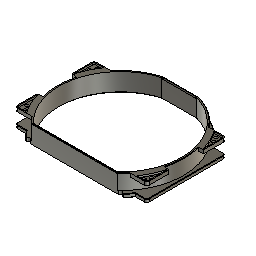
NH-D15 Spacer v9 (Autodesk Fusion 360 design; units mm, degrees)
Autodesk Fusion 360 part; units mm, degrees
sketch "Core" plane through (0, 0, 0) normal (0, 0, 1) x (1, 0, 0)
  line L0 (-49.3785, -52.4) -> (0, -52.4)
  line L1 (0, 69) -> (-20.567, 69)
  line L2 (0, 67) -> (-20.2731, 67)
  line L3 (0, -50) -> (-48.9898, -50)
  arc A0 (-20.2731, 67) -> (-48.9898, -50) centre (0, 0) ccw
  arc A1 (-20.567, 69) -> (-49.3785, -52.4) centre (0, 0) ccw
  line L4 (0, -50) -> (0, 0)
  line L5 (0, 0) -> (0, 67)
  line L6 (0, 67) -> (0, 69)
  line L7 (0, -50) -> (0, -52.4)
  line L8 (0, 69) -> (20.567, 69)
  arc A2 (49.3785, -52.4) -> (20.567, 69) centre (0, 0) ccw
  line L9 (49.3785, -52.4) -> (0, -52.4)
  line L10 (0, 67) -> (20.2731, 67)
  arc A3 (48.9898, -50) -> (20.2731, 67) centre (0, 0) ccw
  line L11 (0, -50) -> (48.9898, -50)
  dimension "d8" = 70
  dimension "d9" = 72
  dimension "d27" = 2
  dimension "d28" = 2.4
  dimension "d29" = 67
  dimension "d30" = 50
  constraint coincident A0.centre A1.centre
  constraint horizontal L3
  constraint horizontal L1
  constraint horizontal L2
  constraint horizontal L0
  constraint vertical L5
  constraint vertical L4
  constraint perpendicular L2 L6
  constraint perpendicular L0 L7
  constraint symmetric L3.start L5 L4.start
  constraint symmetric L0.start L5 A2.start
  constraint symmetric L3.end L5 A3.start
  constraint symmetric L1.end L5 L8.end
  constraint symmetric L2.start L5 L6.start
  constraint symmetric L2.end L5 L10.end
  constraint symmetric L0.end L5 L7.end
  constraint symmetric L1.start L5 L6.end
  constraint symmetric A0 L5 A3
  constraint symmetric A1 L5 A2
  measures "d8" radius of A0
  measures "d9" radius of A1
  measures "d27" distance of L1 L2
  measures "d28" distance of L0 L3
  measures "d29" vertical distance of L2.start A0.centre
  measures "d30" vertical distance of L3.start A0.centre
extrude "Extrude1" add sketch "Core" along normal blind 21 contours L0 L1 L2 L3 A0 A1 L6 L7 | L6 L7 L8 A2 L9 L10 A3 L11
sketch "Base" plane through (0, 0, 0) normal (0, 0, 1) x (1, 0, 0)
  line L0 (-31.3986, 69.7594) -> (0, 69.7594)
  line L1 (-72, 45) -> (-61.8648, 45)
  line L2 (-50.5025, -52.4) -> (-49.3785, -52.4)
  line L3 (-54.4975, -52.4) -> (-55.7359, -52.4)
  line L4 (-75, 42) -> (-75, -42)
  line L5 (-72, -45) -> (-61.8648, -45)
  line L6 (0, 0) -> (0, 67)
  line L7 (0, 69) -> (-20.567, 69)
  arc A0 (-20.567, 69) -> (-49.3785, -52.4) centre (0, 0) ccw
  line L8 (0, 69) -> (0, 69.7594)
  circle A1 centre (-52.5, 52.5) radius 2
  arc A2 (-21.8524, 73.3125) -> (-52.4647, -55.675) centre (0, 0) ccw
  circle A3 centre (-52.5, 52.5) radius 4.5
  circle A4 centre (-52.5, -52.5) radius 2
  arc A5 (-72, 45) -> (-75, 42) centre (-72, 42) ccw
  arc A6 (-75, -42) -> (-72, -45) centre (-72, -42) ccw
  arc A7 (49.3785, -52.4) -> (20.567, 69) centre (0, 0) ccw
  arc A8 (52.4647, -55.675) -> (21.8524, 73.3125) centre (0, 0) ccw
  line L9 (54.4975, -52.4) -> (55.7359, -52.4)
  line L10 (75, 42) -> (75, -42)
  line L11 (72, -45) -> (61.8648, -45)
  circle A9 centre (52.5, 52.5) radius 4.5
  arc A10 (75, 42) -> (72, 45) centre (72, 42) ccw
  line L12 (50.5025, -52.4) -> (49.3785, -52.4)
  circle A11 centre (52.5, 52.5) radius 2
  line L13 (72, 45) -> (61.8648, 45)
  circle A12 centre (52.5, -52.5) radius 2
  arc A13 (72, -45) -> (75, -42) centre (72, -42) ccw
  line L14 (0, 69) -> (20.567, 69)
  line L15 (31.3986, 69.7594) -> (0, 69.7594)
  point P0 (0, 67)
  dimension "d31" = 0.7594
  dimension "d40" = 75
  dimension "d43" = 4
  dimension "d44" = 52.5
  dimension "d45" = 52.5
  dimension "d46" = 4.5
  dimension "d47" = 9
  dimension "d64" = 4
  dimension "d65" = 52.5
  dimension "d66" = 52.5
  dimension "d67" = 90
  dimension "d69" = 45
  dimension "d71" = 84
  dimension "d72" = 42
  constraint coincident L7.start L8.start
  constraint perpendicular L0 L8
  constraint parallel L0 L7
  constraint horizontal L1
  constraint vertical L4
  constraint horizontal L2
  constraint horizontal L3
  constraint collinear L2 L3
  constraint parallel L1 L5
  constraint coincident A2 L0.start
  constraint concentric A1 A3
  constraint coincident A2 L1.end
  constraint coincident A2 L5.end
  constraint coincident L3.end A2
  constraint tangent L4 A5
  constraint tangent L5 A6
  constraint tangent L4 A6
  constraint tangent L1 A5
  constraint symmetric L4.start L6 L10.start
  constraint symmetric L4.end L6 L10.end
  constraint symmetric L1.start L6 A10.end
  constraint symmetric L2.start L6 L12.start
  constraint symmetric L5.start L6 L11.start
  constraint symmetric L3.start L6 L9.start
  constraint symmetric L0.end L6 L8.end
  constraint symmetric L3.end L6 L9.end
  constraint symmetric L6 L7.start L8.start
  constraint symmetric L6 L7.end A7.end
  constraint symmetric L6 L2.end A7.start
  constraint symmetric L6 A0 A7
  constraint symmetric L6 A1 A11
  constraint symmetric L6 A2.end A8.start
  constraint symmetric L6 A2.start A8.end
  constraint symmetric L6 A2 A8
  constraint symmetric L6 L0.start L15.start
  constraint symmetric L6 A3 A9
  constraint symmetric L6 L1.end L13.end
  constraint symmetric L6 L5.end L11.end
  constraint symmetric L6 A4 A12
  constraint symmetric L6 A5 A10
  constraint symmetric L6 A6 A13
  measures "d31" distance of L0 L7
  measures "d40" distance of L4 L6
  measures "d43" diameter of A1
  measures "d44" distance of L6 A1.centre
  measures "d45" vertical distance of L6.start A1.centre
  measures "d47" diameter of A3
  measures "d64" diameter of A4
  measures "d65" horizontal distance of L6.start A4.centre
  measures "d66" vertical distance of L6.start A4.centre
  measures "d67" distance of L1 L5
  measures "d69" distance of L6.start L1
  measures "d71" distance of L4.start L4.end
  measures "d72" vertical distance of L4.start L6.start
extrude "Extrude2" add sketch "Base" along normal blind 4 contours L0 L7 A0 L8 A2 A3 | L8 A7 A8 A9 L14 L15 | A0 A2 A3 | A2 A3 | L2 L3 L4 A0 A2 A3 A4 | A8 A9 | A7 A8 A9 | L1 L4 A2 A5 | A7 A8 L9 L10 A9 L12 A12 | A8 L10 A10 L13 | L4 L5 A2 A6 | A8 L10 L11 A13
ref_plane "WorkPlane3" through (0, 0, 21) normal (0, 0, 1) x (1, 0, 0)
sketch "Top" plane through (0, 0, 21) normal (0, 0, 1) x (1, 0, 0)
  line L0 (-73.9, 42) -> (-73.9, 20.9955)
  circle A0 centre (-70.9, 35.5) radius 1.8
  circle A1 centre (-67.9, 41) radius 1.8
  line L1 (-75, 20) -> (-69.4423, 19.02)
  line L2 (-73.9, 20.9955) -> (-73.5786, 20.9388)
  line L3 (-72, 43.9) -> (-62.8, 43.9)
  line L4 (-62.8, 43.9) -> (-62.8, 43.6854)
  line L5 (0, 0) -> (-10, 0)
  line L6 (-72, 45) -> (-61.8648, 45)
  arc A2 (-72, 45) -> (-75, 42) centre (-72, 42) ccw
  line L7 (-75, 42) -> (-75, -42)
  line L8 (-75, 20) -> (-75, 42)
  line L9 (-72, 45) -> (-56.205, 45)
  arc A3 (-21.8524, 73.3125) -> (-52.4647, -55.675) centre (0, 0) ccw
  arc A4 (-20.567, 69) -> (-49.3785, -52.4) centre (0, 0) ccw
  arc A5 (-72, 43.9) -> (-73.9, 42) centre (-72, 42) ccw
  arc A6 (-62.8, 43.6853) -> (-73.5786, 20.9388) centre (0, 0) ccw
  arc A7 (-56.205, 45) -> (-69.4423, 19.02) centre (0, 0) ccw
  line L10 (0, 0) -> (0, 67)
  line L11 (-75, -20) -> (-75, -42)
  line L12 (-73.9, -20.9955) -> (-73.5786, -20.9388)
  line L13 (-72, -43.9) -> (-62.8, -43.9)
  line L14 (-62.8, -43.9) -> (-62.8, -43.6853)
  arc A8 (-73.9, -42) -> (-72, -43.9) centre (-72, -42) ccw
  circle A9 centre (-67.9, -41) radius 1.8
  line L15 (-72, -45) -> (-61.8648, -45)
  circle A10 centre (-70.9, -35.5) radius 1.8
  line L16 (-75, -20) -> (-69.4423, -19.02)
  arc A11 (-73.5786, -20.9388) -> (-62.8, -43.6853) centre (0, 0) ccw
  line L17 (-72, -45) -> (-56.205, -45)
  arc A12 (-69.4423, -19.02) -> (-56.205, -45) centre (0, 0) ccw
  arc A13 (-75, -42) -> (-72, -45) centre (-72, -42) ccw
  line L18 (-73.9, -42) -> (-73.9, -20.9955)
  line L19 (62.8, -43.9) -> (62.8, -43.6853)
  circle A14 centre (67.9, 41) radius 1.8
  line L20 (73.9, -20.9955) -> (73.5786, -20.9388)
  line L21 (75, -20) -> (69.4423, -19.02)
  arc A15 (62.8, -43.6853) -> (73.5786, -20.9388) centre (0, 0) ccw
  line L22 (73.9, -42) -> (73.9, -20.9955)
  line L23 (72, -45) -> (56.205, -45)
  line L24 (73.9, 20.9955) -> (73.5786, 20.9388)
  arc A16 (73.5786, 20.9388) -> (62.8, 43.6853) centre (0, 0) ccw
  line L25 (72, -43.9) -> (62.8, -43.9)
  circle A17 centre (67.9, -41) radius 1.8
  line L26 (72, 43.9) -> (62.8, 43.9)
  arc A18 (75, 42) -> (72, 45) centre (72, 42) ccw
  line L27 (72, 45) -> (56.205, 45)
  arc A19 (73.9, 42) -> (72, 43.9) centre (72, 42) ccw
  arc A20 (72, -45) -> (75, -42) centre (72, -42) ccw
  line L28 (75, -20) -> (75, -42)
  arc A21 (56.205, -45) -> (69.4423, -19.02) centre (0, 0) ccw
  arc A22 (72, -43.9) -> (73.9, -42) centre (72, -42) ccw
  arc A23 (69.4423, 19.02) -> (56.205, 45) centre (0, 0) ccw
  line L29 (72, 45) -> (61.8648, 45)
  line L30 (62.8, 43.9) -> (62.8, 43.6853)
  line L31 (73.9, 42) -> (73.9, 20.9955)
  circle A24 centre (70.9, -35.5) radius 1.8
  line L32 (75, 20) -> (69.4423, 19.02)
  circle A25 centre (70.9, 35.5) radius 1.8
  line L33 (72, -45) -> (61.8648, -45)
  line L34 (75, 20) -> (75, 42)
  point P0 (-72, 41.9955)
  point P1 (-75, -42)
  point P2 (-72, -41.9955)
  point P3 (75, -42)
  point P4 (75, -42)
  point P5 (75, 42)
  point P6 (72, -41.9955)
  point P7 (72, 41.9955)
  dimension "d76" = 22
  dimension "d77" = 100
  dimension "d78" = -1.1
  dimension "d79" = 2.9
  dimension "d80" = 3
  dimension "d81" = 8.4
  dimension "d82" = 6
  dimension "d84" = 0.3263
  dimension "d85" = 3.6
  dimension "d86" = 3.6
  dimension "d89" = 9.2
  constraint coincident A2.end L7.start
  constraint tangent A2 L8
  constraint coincident L6.start A2.start
  constraint tangent A2 L9
  constraint perpendicular L8 L9
  constraint coincident A4 L9.end
  constraint coincident A4 L1.end
  constraint parallel L1 L2
  constraint parallel L0 L8
  constraint parallel L3 L9
  constraint tangent L3 A5
  constraint tangent L0 A5
  constraint perpendicular L3 L4
  constraint coincident A3 A6.start
  constraint coincident A3 L2.end
  constraint symmetric P0 L5 P2
  constraint symmetric L5 L3.start L13.start
  constraint symmetric L3.end L5 L13.end
  constraint symmetric L0.end L5 L12.start
  constraint symmetric L1.start L5 L11.start
  constraint symmetric L5 L0.start A8.start
  constraint symmetric A0 L5 A10
  constraint symmetric A1 L5 A9
  constraint symmetric L5 L6.start L15.start
  constraint symmetric L5 L6.end L15.end
  constraint symmetric L5 A2.end P1
  constraint symmetric L5 A2 A13
  constraint symmetric L5 L9.end L17.end
  constraint symmetric L5 L1.end L16.end
  constraint symmetric L5 A5 A8
  constraint symmetric L5 A6.start L14.end
  constraint symmetric L5 L2.end L12.end
  constraint symmetric L5 A6 A11
  constraint symmetric L5 A7 A12
  constraint symmetric P0 L10 P7
  constraint symmetric L3.start L10 L26.start
  constraint symmetric L3.end L10 L26.end
  constraint symmetric L0.end L10 L24.start
  constraint symmetric L1.start L10 L32.start
  constraint symmetric L0.start L10 A19.start
  constraint symmetric A0 L10 A25
  constraint symmetric A1 L10 A14
  constraint symmetric L6.start L10 A18.end
  constraint symmetric L6.end L10 L29.end
  constraint symmetric A2.end L10 P5
  constraint symmetric A2 L10 A18
  constraint symmetric P1 L10 P4
  constraint symmetric L9.end L10 L27.end
  constraint symmetric L1.end L10 A23.start
  constraint symmetric A5 L10 A19
  constraint symmetric A6.start L10 A16.end
  constraint symmetric L2.end L10 L24.end
  constraint symmetric A6 L10 A16
  constraint symmetric A7 L10 A23
  constraint symmetric L10 P1 P4
  constraint symmetric L10 L15.start L23.start
  constraint symmetric L10 L13.end L19.start
  constraint symmetric L10 L13.start L25.start
  constraint symmetric L10 L12.start L20.start
  constraint symmetric L10 L11.start L21.start
  constraint symmetric L10 A8.start L22.start
  constraint symmetric L10 L15.end L33.end
  constraint symmetric L10 L14.end L19.end
  constraint symmetric L10 L17.end L23.end
  constraint symmetric L10 P2 P6
  constraint symmetric L10 L12.end L20.end
  constraint symmetric L10 A8 A22
  constraint symmetric L10 A9 A17
  constraint symmetric L10 A10 A24
  constraint symmetric L10 L16.end L21.end
  constraint symmetric L10 A11 A15
  constraint symmetric L10 A12 A21
  constraint symmetric L10 A13 A20
  constraint coincident A3 L4.end
  measures "d76" distance of L1.start A2.end
  measures "d77" angle of L1 L8
  measures "d79" distance of A1.centre L3
  measures "d80" distance of A0.centre L0
  measures "d81" distance of A0.centre L3
  measures "d82" distance of A1.centre L0
  measures "d84" distance of L0.end L2.end
  measures "d85" diameter of A0
  measures "d86" diameter of A1
  measures "d89" distance of L3.end L3.start
extrude "Extrude5" add sketch "Top" against normal blind 4 contours L0 L2 L3 L4 A3 A5 A6 | L0 L1 L2 L3 L4 L6 A2 L7 L8 L9 A3 A5 | L1 L9 A3 A4 A6 A7 | A3 A4 L16 A11 L17 A12 | L7 A3 L11 L12 L13 L14 A8 L15 L16 L17 A13 L18 | A3 L12 L13 L14 A8 A11 L18 | L19 L20 A15 L22 L25 A22 | L21 L23 A20 L28 A21 L33 | L24 A16 L26 A19 L30 L31 | A18 L27 A23 L29 L32 L34
extrude "Extrude6" cut sketch "Top" against normal blind 2 contours L0 L2 L3 L4 A3 A5 A6 | A3 L12 L13 L14 A8 A11 L18 | L19 L20 A15 L22 L25 A22 | L24 A16 L26 A19 L30 L31
chamfer "Chamfer1" distance 0.5 angle 45 52 edges at (-40.2179, 59.7203, 21) (-72, 0, 21) (-75, 0, 4) (-74.1213, 44.1213, 4) (-66.9324, 45, 4) (-66.9324, -45, 4) (-74.1213, -44.1213, 4) (-59.4221, 48.1795, 4) (-55.682, 55.682, 4) (-41.8165, 64.0596, 4) (-41.8165, 64.0596, 0) (-55.682, 55.682, 0) (-59.4221, 48.1795, 0) (-75, 0, 0) (-74.1213, 44.1213, 0) (-66.9324, 45, 0) (-66.9324, -45, 0) (-74.1213, -44.1213, 0) (-58.9166, -48.7963, 4) (-58.9166, -48.7963, 0) (-52.9213, -48.8195, 21) (-55.1167, -52.4, 4) (-55.1167, -52.4, 0) (-49.9405, -52.4, 4) (0, -52.4, 0) (0, -52.4, 21) (49.9405, -52.4, 4) (55.1167, -52.4, 4) (55.1167, -52.4, 0) (58.9166, -48.7963, 0) (58.9166, -48.7963, 4) (66.9324, -45, 4) (74.1213, -44.1213, 4) (75, 0, 4) (74.1213, 44.1213, 4) (66.9324, 45, 4) (66.9324, -45, 0) (74.1213, -44.1213, 0) (75, 0, 0) (74.1213, 44.1213, 0) (66.9324, 45, 0) (72, 0, 21) (41.8165, 64.0596, 4) (41.8165, 64.0596, 0) (59.4221, 48.1795, 0) (59.4221, 48.1795, 4) (55.682, 55.682, 4) (55.682, 55.682, 0) (0, 69.7594, 4) (0, 69.7594, 0) (40.2179, 59.7203, 21) (0, 69, 21)
chamfer "Chamfer1" distance 0.5 angle 45 1 edges at (52.9213, -48.8195, 21)
chamfer "Chamfer2" distance 1 angle 45 6 edges at (0, -50, 0) (0, 67, 0) (67.9823, 16.6857, 0) (-67.9823, 16.6857, 0) (0, -50, 21) (0, 67, 21)
named bodies: "Core"
